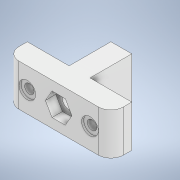
# Autodesk Inventor part: Z_item_mount
Saved by Autodesk Inventor 2020 (Build 240168000, 168)
## iProperties
Created: 2022-03-24
Part Number: Z_item_mount
Material: Tworzywo sztuczne ABS
Document SubType Name: Modeling
Designer: mikoma
Density: 1.06 g/cm^3
Appearance: Gładki — biały
Mass: 12.3763 g
Surface Area: 54.2984 cm^2
Volume: 11.6758 cm^3
Author: mikoma
Autodesk Inventor part; units mm, degrees
ref_plane "YZ Plane" through (0, 0, 0) normal (1, 0, 0) x (0, 1, 0)
ref_plane "XZ Plane" through (0, 0, 0) normal (0, 1, 0) x (-1, 0, 0)
ref_plane "XY Plane" through (0, 0, 0) normal (0, 0, 1) x (1, 0, 0)
sketch "Szkic1" plane through (0, 0, 0) normal (0, 1, 0) x (-1, 0, 0)
  line L0 (25, 20) -> (5, 20)
  line L1 (5, 20) -> (5, 0)
  line L2 (5, 0) -> (25, 0)
  line L3 (25, 0) -> (25, 20)
  line L4 (-5, 20) -> (-25, 20)
  line L5 (-25, 20) -> (-25, 0)
  line L6 (-25, 0) -> (-5, 0)
  line L7 (-5, 0) -> (-5, 20)
  line L8 (25, 0) -> (-25, 0)
  line L9 (-25, 0) -> (-25, 30)
  line L10 (-25, 30) -> (25, 30)
  line L11 (25, 30) -> (25, 0)
  point P0 (0, 0)
  point P1 (-15, 20)
  point P2 (15, 20)
  point P3 (15, 0)
  point P4 (-5, 0)
  point P5 (5, 0)
  dimension "d0" = 20
  dimension "d1" = 20
  dimension "d2" = 20
  dimension "d3" = 20
  dimension "d4" = 50
  dimension "d5" = 25
  dimension "d6" = 10
  constraints: 24 end point, 6 parallel, 3 horizontal, 3 midpoint, 3 perpendicular, 2 horizontal alignment, 1 vertical alignment
  measures "d0" distance of L2.end L0.start
  measures "d1" distance of L1.end L2.end
  measures "d2" distance of L6.end L4.start
  measures "d3" distance of L5.end L6.end
  measures "d4" distance between parallel lines of L5 L3
  measures "d5" distance from line of point (0, 0) L3
  measures "d6" distance between parallel lines of L0 L10
extrude "Wyciągnięcie proste1" add sketch "Szkic1" along normal blind 20 contours L0 L1 L8 L7 L4 L9 L10 L11
sketch "Szkic2" plane through (5, 0, 0) normal (0, 0, -1) x (-1, 0, 0)
  circle A0 centre (5, 10) radius 3.25
  circle A1 centre (20, 10) radius 2.25
  circle A2 centre (-10, 10) radius 2.25
  line L0 (0, 0) -> (0, 20) projected
  line L1 (0, 0) -> (10, 0) projected
  line L2 (-20, 0) -> (-20, 20) projected
  line L3 (-20, 0) -> (0, 0) projected
  line L4 (30, 0) -> (30, 20) projected
  circle A3 centre (-10, 10) radius 4
  circle A4 centre (20, 10) radius 4
  line L5 (1.8246, 15.5) -> (8.1754, 15.5)
  line L6 (8.1754, 15.5) -> (11.3509, 10)
  line L7 (11.3509, 10) -> (8.1754, 4.5)
  line L8 (8.1754, 4.5) -> (1.8246, 4.5)
  line L9 (1.8246, 4.5) -> (-1.3509, 10)
  line L10 (-1.3509, 10) -> (1.8246, 15.5)
  point P0 (5, 0)
  dimension "d9" = 6.5
  dimension "d10" = 5
  dimension "d11" = 10
  dimension "d12" = 10
  dimension "d13" = 10
  dimension "d14" = 10
  dimension "d15" = 4.5
  dimension "d16" = 4.5
  dimension "d20" = 8
  dimension "d21" = 8
  dimension "d25" = 11
  constraints: 12 end point, 5 centre point, 3 coincident, 1 horizontal, 1 horizontal alignment, 13 other
  measures "d9" diameter of A0
  measures "d10" distance from line of A0.centre L0
  measures "d11" distance from line of L1 A0.centre
  measures "d12" distance from line of L2 A2.centre
  measures "d13" distance from line of A2.centre L3
  measures "d14" distance from line of L4 A1.centre
  measures "d15" diameter of A2
  measures "d16" diameter of A1
  measures "d20" diameter of A3
  measures "d21" diameter of A4
  measures "d25" distance between parallel lines of L8 L5
extrude "Wyciągnięcie proste2" cut sketch "Szkic2" against normal through all contours A0 | A1 | A2
extrude "Wyciągnięcie proste3" cut sketch "Szkic2" along normal blind 5 from surface at -30 contours A0 | L9 L10 L0 | L0 L10 L5 L6 L7 L8 L9
fillet "Zaokrąglenie1" radius 6 2 edges at (25, 10, 30) (-25, 10, 30)
extrude "Wyciągnięcie proste4" cut sketch "Szkic2" along normal blind 1 from surface at -30 contours A1 | A2 | A3 | A4
